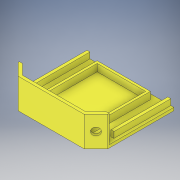
# Autodesk Inventor part: bottom-housing
Saved by Autodesk Inventor 2018 (Build 220112000, 112)
## iProperties
Created: 2019-10-14
Part Number: bottom-housing
Material: Generic
Document SubType Name: Modeling
Designer: jklei
Density: 1 g/cm^3
Appearance: Default
Author: jklei
Autodesk Inventor part; units mm, degrees
ref_plane "YZ Plane" through (0, 0, 0) normal (1, 0, 0) x (0, 1, 0)
ref_plane "XZ Plane" through (0, 0, 0) normal (0, 1, 0) x (-1, 0, 0)
ref_plane "XY Plane" through (0, 0, 0) normal (0, 0, 1) x (1, 0, 0)
sketch "Sketch1" plane through (0, 0, 0) normal (0, 1, 0) x (-1, 0, 0)
  line L0 (0, 0) -> (95.25, 0)
  line L1 (95.25, 0) -> (95.25, -82.55)
  line L2 (95.25, -82.55) -> (0, -82.55)
  line L3 (0, -82.55) -> (0, 0)
  dimension "d0" = 95.25
  dimension "d1" = 82.55
  constraints: 8 end point, 2 parallel, 1 horizontal, 1 perpendicular
  measures "d0" distance of L1.end L2.end
  measures "d1" distance of L0.end L1.end
extrude "Extrusion1" add sketch "Sketch1" along normal blind 3.175
chamfer "Chamfer1" distance 12.7 angle 45 2 edges at (-95.25, 1.5875, 0) (0, 1.5875, 0)
sketch "Sketch9" plane through (0, 3.175, 0) normal (0, 1, 0) x (1, 0, 0)
  line L0 (0, 12.7) -> (-12.7, 0) projected
  line L1 (0, 12.7) -> (0, 82.55) projected
  line L2 (0, 82.55) -> (-95.25, 82.55) projected
  line L3 (-95.25, 82.55) -> (-95.25, 12.7) projected
  line L4 (-82.55, 0) -> (-95.25, 12.7) projected
  line L5 (-82.55, 0) -> (-12.7, 0) projected
  line L6 (-3.175, 14.0151) -> (-14.0151, 3.175)
  line L7 (-14.0151, 3.175) -> (-81.2349, 3.175)
  line L8 (-81.2349, 3.175) -> (-92.075, 14.0151)
  line L9 (-95.25, 82.55) -> (0, 82.55) projected
  line L10 (-92.075, 14.0151) -> (-95.25, 14.0151)
  line L11 (-95.25, 12.7) -> (-95.25, 82.55) projected
  line L12 (-3.175, 14.0151) -> (0, 14.0151)
  point P0 (0, 0)
  point P1 (-3.175, 98.425)
  point P2 (-3.175, 82.55)
  dimension "d42" = 68.5349
  constraints: 10 end point, 3 point on line, 2 horizontal, 2 other
  measures "d42" distance between parallel lines of L2 L12
extrude "Extrusion8" add sketch "Sketch9" along normal blind 28.575 contours L0 L5 L4 L3 L10 L8 L7 L6 L12 L1
sketch "Sketch12" plane through (0, 3.175, 0) normal (0, 1, 0) x (1, 0, 0)
  line L0 (0, 82.55) -> (-95.25, 82.55) projected
  line L1 (0, 82.55) -> (-3.175, 82.55)
  line L2 (-14.0151, 3.175) -> (-3.175, 14.0151) projected
  line L3 (-3.175, 82.55) -> (-6.35, 82.55)
  line L4 (-6.35, 82.55) -> (-6.35, 22.225)
  line L5 (-6.35, 22.225) -> (-3.175, 22.225)
  line L6 (-3.175, 22.225) -> (-3.175, 82.55)
  line L7 (-95.25, 82.55) -> (-92.075, 82.55)
  line L8 (-92.075, 82.55) -> (-88.9, 82.55)
  line L9 (-88.9, 82.55) -> (-88.9, 22.225)
  line L10 (-88.9, 22.225) -> (-92.075, 22.225)
  line L11 (-92.075, 22.225) -> (-92.075, 82.55)
  point P0 (0, 0)
  point P1 (0, 17.1901)
  dimension "d34" = 3.175
  dimension "d35" = 3.175
  dimension "d36" = 60.325
  dimension "d37" = 3.175
  dimension "d38" = 3.175
  dimension "d39" = 60.325
  constraints: 20 end point, 4 parallel, 2 horizontal, 2 perpendicular, 2 point on line
  measures "d34" distance of L0.start L1.end
  measures "d35" distance of L5.end L4.end
  measures "d36" distance of L4.end L3.end
  measures "d37" distance of L0.end L7.end
  measures "d38" distance of L9.end L10.end
  measures "d39" distance of L8.end L9.end
extrude "Extrusion10" add sketch "Sketch12" along normal blind 6.35
sketch "Sketch13" plane through (-12.7, 0, 0) normal (0.7071068, 0, 0.7071068) x (0.7071068, 0, -0.7071068)
  line L0 (0, 31.75) -> (0, 0) projected
  line L1 (0, 15.875) -> (17.824, 15.875)
  circle A0 centre (8.912, 15.875) radius 4.15
  point P0 (8.9803, 0)
  point P1 (0, 3.175)
  dimension "d43" = 8.3
  constraints: 2 end point, 2 midpoint, 1 centre point, 1 horizontal
  measures "d43" diameter of A0
extrude "Extrusion11" cut sketch "Sketch13" against normal up to next
sketch "Sketch14" plane through (-95.25, 0, -12.7) normal (-0.7071068, 0, 0.7071068) x (0.7071068, 0, 0.7071068)
  line L0 (17.9605, 0) -> (17.9605, 31.75) projected
  line L1 (17.9605, 15.875) -> (0, 15.875)
  line L2 (0, 31.75) -> (0, 0) projected
  circle A0 centre (8.9803, 15.875) radius 4.15
  point P0 (76.3322, 0)
  point P1 (17.9605, 3.175)
  point P2 (0, 3.175)
  dimension "d46" = 8.3
  constraints: 3 midpoint, 2 end point, 1 centre point
  measures "d46" diameter of A0
extrude "Extrusion12" cut sketch "Sketch14" against normal up to next
sketch "Sketch15" plane through (0, 3.175, 0) normal (0, 1, 0) x (1, 0, 0)
  line L0 (-73.025, 74.295) -> (-22.225, 74.295)
  line L1 (-22.225, 74.295) -> (-22.225, 9.525)
  line L2 (-22.225, 9.525) -> (-73.025, 9.525)
  line L3 (-73.025, 9.525) -> (-73.025, 74.295)
  line L4 (-6.35, 22.225) -> (-6.35, 82.55) projected
  line L5 (0, 12.7) -> (0, 82.55) projected
  line L6 (-21.971, 74.549) -> (-73.279, 74.549)
  line L7 (-73.279, 74.549) -> (-73.279, 9.271)
  line L8 (-73.279, 9.271) -> (-21.971, 9.271)
  line L9 (-21.971, 9.271) -> (-21.971, 74.549)
  line L10 (-75.819, 77.089) -> (-19.431, 77.089)
  line L11 (-19.431, 77.089) -> (-19.431, 6.731)
  line L12 (-19.431, 6.731) -> (-75.819, 6.731)
  line L13 (-75.819, 6.731) -> (-75.819, 77.089)
  line L14 (-14.0151, 3.175) -> (-81.2349, 3.175) projected
  point P0 (0, 0)
  point P1 (0, 14.0151)
  point P2 (0, 17.1901)
  point P3 (-6.35, 10.8401)
  dimension "d49" = 50.8
  dimension "d50" = 64.77
  dimension "d52" = 22.225
  dimension "d53" = 0.254
  dimension "d54" = 2.54
  dimension "d57" = 6.35
  constraints: 24 end point, 6 parallel, 3 perpendicular, 1 horizontal, 6 other
  measures "d49" distance of L1.end L2.end
  measures "d50" distance of L0.end L1.end
  measures "d52" distance between parallel lines of L5 L1
  measures "d53" distance between parallel lines of L0 L6
  measures "d54" distance between parallel lines of L6 L10
  measures "d57" distance between parallel lines of L14 L2
extrude "Extrusion13" add sketch "Sketch15" along normal blind 7.62 contours L10 L11 L12 L13
body "Solid1"
